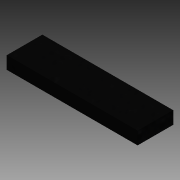
# Autodesk Inventor part: GPIO_conector
Saved by Autodesk Inventor 2015 (Build 190159000, 159)
## iProperties
Created: 2016-01-04
Part Number: GPIO_conector
Material: Generic
Document SubType Name: Modeling
Designer: david
Density: 1 g/cm^3
Appearance: Fine Textured - Black
Author: david
Autodesk Inventor part; units mm, degrees
ref_plane "YZ Plane" through (0, 0, 0) normal (1, 0, 0) x (0, 1, 0)
ref_plane "XZ Plane" through (0, 0, 0) normal (0, 1, 0) x (-1, 0, 0)
ref_plane "XY Plane" through (0, 0, 0) normal (0, 0, 1) x (1, 0, 0)
sketch "Sketch1" plane through (0, 0, 0) normal (0, 1, 0) x (-1, 0, 0)
  line L0 (-25.75, -2.5) -> (25.75, -2.5)
  line L1 (25.75, -2.5) -> (25.75, 2.5)
  line L2 (25.75, 2.5) -> (-25.75, 2.5)
  line L3 (-25.75, 2.5) -> (-25.75, -2.5)
  line L4 (-25.75, -2.5) -> (25.75, 2.5) construction
  line L5 (25.75, -2.5) -> (-25.75, 2.5) construction
  point P0 (0, 0)
  dimension "d0" = 51.5
  dimension "d1" = 5
  constraints: 12 end point, 2 midpoint, 2 parallel, 1 horizontal, 1 perpendicular
  measures "d0" distance of L2.end L1.end
  measures "d1" distance of L1.end L0.end
extrude "Extrusion1" add sketch "Sketch1" along normal blind 14
body "Solid1"
